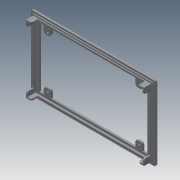
# Autodesk Inventor part: lower
Saved by Autodesk Inventor 2014 (Build 180170000, 170)
## iProperties
Created: 2014-09-06
Part Number: lower
Material: 一般
Document SubType Name: Modeling
Designer: Hideyuki Takei
Density: 1 g/cm^3
Appearance: 既定
Author: Hideyuki Takei
Autodesk Inventor part; units mm, degrees
ref_plane "YZ Plane" through (0, 0, 0) normal (1, 0, 0) x (0, 1, 0)
ref_plane "XZ Plane" through (0, 0, 0) normal (0, 1, 0) x (-1, 0, 0)
ref_plane "XY Plane" through (0, 0, 0) normal (0, 0, 1) x (1, 0, 0)
sketch "スケッチ2" plane through (0, 0, 0) normal (0, 1, 0) x (-1, 0, 0)
  line L0 (0, 0) -> (136, 0)
  line L1 (136, 0) -> (136, 81)
  line L2 (136, 81) -> (0, 81)
  line L3 (0, 81) -> (0, 0)
  dimension "d2" = 81
  dimension "d3" = 136
  constraints: 8 end point, 2 parallel, 1 horizontal, 1 perpendicular
  measures "d2" distance of L2.end L0.start
  measures "d3" distance of L1.end L2.end
extrude "押し出し1" add sketch "スケッチ2" along normal blind 2
sketch "スケッチ3" plane through (0, 0, 0) normal (0, 1, 0) x (-1, 0, 0)
  line L0 (5, 5) -> (131, 5)
  line L1 (131, 5) -> (131, 76)
  line L2 (131, 76) -> (5, 76)
  line L3 (5, 76) -> (5, 5)
  line L4 (136, 0) -> (136, 81) projected
  line L5 (136, 81) -> (0, 81) projected
  line L6 (132.5, 77.5) -> (126.5, 77.5)
  line L7 (126.5, 77.5) -> (126.5, 76)
  line L8 (126.5, 76) -> (132.5, 76)
  line L9 (132.5, 76) -> (132.5, 77.5)
  line L10 (131, 76) -> (132.5, 76)
  line L11 (132.5, 76) -> (132.5, 71)
  line L12 (132.5, 71) -> (131, 71)
  line L13 (131, 71) -> (131, 76)
  line L14 (131, 5) -> (132.5, 5)
  line L15 (132.5, 5) -> (132.5, 10)
  line L16 (132.5, 10) -> (131, 10)
  line L17 (131, 10) -> (131, 5)
  line L18 (132.5, 5) -> (126.5, 5)
  line L19 (126.5, 5) -> (126.5, 3.5)
  line L20 (126.5, 3.5) -> (132.5, 3.5)
  line L21 (132.5, 3.5) -> (132.5, 5)
  line L22 (5, 76) -> (3.5, 76)
  line L23 (3.5, 76) -> (3.5, 71)
  line L24 (3.5, 71) -> (5, 71)
  line L25 (5, 71) -> (5, 76)
  line L26 (3.5, 76) -> (9.5, 76)
  line L27 (9.5, 76) -> (9.5, 77.5)
  line L28 (9.5, 77.5) -> (3.5, 77.5)
  line L29 (3.5, 77.5) -> (3.5, 76)
  line L30 (5, 5) -> (3.5, 5)
  line L31 (3.5, 5) -> (3.5, 10)
  line L32 (3.5, 10) -> (5, 10)
  line L33 (5, 10) -> (5, 5)
  line L34 (3.5, 5) -> (9.5, 5)
  line L35 (9.5, 5) -> (9.5, 3.5)
  line L36 (9.5, 3.5) -> (3.5, 3.5)
  line L37 (3.5, 3.5) -> (3.5, 5)
  point P0 (0, 0)
  dimension "d6" = 126
  dimension "d7" = 71
  dimension "d8" = 5
  dimension "d9" = 5
  dimension "d10" = 1.5
  dimension "d11" = 1.5
  dimension "d12" = 5
  dimension "d13" = 6
  dimension "d14" = 0
  dimension "d17" = 1.5
  dimension "d18" = 1.5
  dimension "d19" = 6
  dimension "d20" = 5
  dimension "d21" = 5
  dimension "d22" = 1.5
  dimension "d23" = 1.5
  dimension "d24" = 6
  dimension "d25" = 6
  dimension "d26" = 1.5
  dimension "d27" = 1.5
  dimension "d28" = 5
  constraints: 72 end point, 18 parallel, 9 horizontal, 9 perpendicular, 1 point on line
  measures "d6" distance of L1.end L2.end
  measures "d7" distance of L0.end L1.end
  measures "d8" distance between parallel lines of L4 L1
  measures "d9" distance between parallel lines of L5 L2
  measures "d10" distance of L11.end L12.end
  measures "d11" distance of L8.end L6.start
  measures "d12" distance of L10.end L11.end
  measures "d13" distance of L6.start L6.end
  measures "d14" distance between parallel lines of L11 L9
  measures "d17" distance of L15.end L16.end
  measures "d18" distance of L20.end L14.end
  measures "d19" distance of L19.end L20.end
  measures "d20" distance of L14.end L15.end
  measures "d21" distance of L22.end L23.end
  measures "d22" distance of L23.end L24.end
  measures "d23" distance of L28.end L22.end
  measures "d24" distance of L27.end L28.end
  measures "d25" distance of L35.end L36.end
  measures "d26" distance of L34.end L35.end
  measures "d27" distance of L31.end L32.end
  measures "d28" distance of L30.end L31.end
extrude "押し出し2" add sketch "スケッチ3" against normal blind 9.01 contours L30 L31 L32 L3 | L0 L35 L36 L37 L30 | L0 L14 L21 L20 L19 | L24 L23 L22 L3 | L1 L16 L15 L14 | L22 L29 L28 L27 L2 | L1 L8 L11 L12 | L7 L6 L9 L8 L2
sketch "スケッチ5" plane through (0, 0, 0) normal (0, 1, 0) x (-1, 0, 0)
  line L0 (131, 76) -> (5, 76)
  line L1 (5, 76) -> (5, 5)
  line L2 (5, 5) -> (131, 5)
  line L3 (131, 5) -> (131, 76)
  line L4 (0, 81) -> (0, 0) projected
  line L5 (131, 76) -> (5, 76)
  line L6 (5, 76) -> (5, 77.5)
  line L7 (5, 77.5) -> (131, 77.5)
  line L8 (131, 77.5) -> (131, 76)
  line L9 (131, 5) -> (5, 5)
  line L10 (5, 5) -> (5, 3.5)
  line L11 (5, 3.5) -> (131, 3.5)
  line L12 (131, 3.5) -> (131, 5)
  line L13 (131, 77.5) -> (132.5, 77.5)
  line L14 (132.5, 77.5) -> (132.5, 3.5)
  line L15 (132.5, 3.5) -> (131, 3.5)
  line L16 (131, 3.5) -> (131, 77.5)
  line L17 (5, 77.5) -> (3.5, 77.5)
  line L18 (3.5, 77.5) -> (3.5, 3.5)
  line L19 (3.5, 3.5) -> (5, 3.5)
  line L20 (5, 3.5) -> (5, 77.5)
  dimension "d34" = 126
  dimension "d35" = 71
  dimension "d36" = 5
  dimension "d37" = 5
  dimension "d38" = 1.5
  dimension "d39" = 1.5
  dimension "d40" = 1.5
  dimension "d41" = 1.5
  dimension "d42" = 1.5
  dimension "d43" = 1.5
  constraints: 40 end point, 10 parallel, 5 horizontal, 5 perpendicular
  measures "d34" distance of L0.start L0.end
  measures "d35" distance of L2.end L0.start
  measures "d36" distance from line of L4.end L2
  measures "d37" distance between parallel lines of L4 L1
  measures "d38" distance of L5.end L6.end
  measures "d39" distance of L9.end L10.end
  measures "d40" distance of L14.end L15.end
  measures "d41" distance of L18.end L19.end
  measures "d42" distance between parallel lines of L19 L2
  measures "d43" distance between parallel lines of L18 L1
extrude "押し出し4" add sketch "スケッチ5" against normal blind 2 contours L8 L13 L14 L15 L12 L3 | L0 L6 L7 L8 | L1 L10 L19 L18 L17 L6 | L12 L11 L10 L2
sketch "スケッチ7" plane through (0, 0, 0) normal (0, 1, 0) x (-1, 0, 0)
  line L0 (9, 73.5) -> (127, 73.5)
  line L1 (127, 73.5) -> (127, 7.5)
  line L2 (127, 7.5) -> (9, 7.5)
  line L3 (9, 7.5) -> (9, 73.5)
  line L4 (136, 0) -> (136, 81) projected
  line L5 (136, 81) -> (0, 81) projected
  point P0 (0, 0)
  dimension "d50" = 66
  dimension "d51" = 118
  dimension "d52" = 9
  dimension "d53" = 7.5
  constraints: 8 end point, 2 parallel, 1 horizontal, 1 perpendicular
  measures "d50" distance of L0.end L1.end
  measures "d51" distance of L1.end L2.end
  measures "d52" distance between parallel lines of L1 L4
  measures "d53" distance between parallel lines of L5 L0
extrude "押し出し6" cut sketch "スケッチ7" along normal up to next
sketch "スケッチ9" plane through (-132.5, 0, 77.5) normal (0, 0, 1) x (1, 0, 0)
  line L0 (129, 0) -> (129, -9.01) projected
  line L1 (0, 0) -> (129, 0) projected
  line L2 (0, 0) -> (129, 0)
  line L3 (129, 0) -> (129, -1)
  line L4 (129, -1) -> (0, -1)
  line L5 (0, -1) -> (0, 0)
  point P0 (132.5, 0)
  dimension "d62" = 1
  constraints: 8 end point, 2 parallel, 1 horizontal, 1 perpendicular, 1 point on line
  measures "d62" distance of L4.end L1.start
extrude "押し出し8" add sketch "スケッチ9" along normal blind 1.5
sketch "スケッチ10" plane through (-3.5, 0, 3.5) normal (0, 0, -1) x (-1, 0, 0)
  line L0 (129, 0) -> (129, -9.01) projected
  line L1 (0, 0) -> (129, 0)
  line L2 (129, 0) -> (129, -1)
  line L3 (129, -1) -> (0, -1)
  line L4 (0, -1) -> (0, 0)
  point P0 (-3.5, 0)
  dimension "d65" = 1
  constraints: 8 end point, 2 parallel, 1 horizontal, 1 perpendicular, 1 point on line
  measures "d65" distance of L1.end L2.end
extrude "押し出し9" add sketch "スケッチ10" along normal blind 1.5
sketch "スケッチ11" plane through (-3.5, -9.01, 10) normal (1, 0, 0) x (0, 0, -1)
  line L0 (-69, 9.01) -> (8, 9.01)
  line L1 (8, 9.01) -> (8, 8.01)
  line L2 (8, 8.01) -> (-69, 8.01)
  line L3 (-69, 8.01) -> (-69, 9.01)
  point P0 (10, 9.01)
  constraints: 8 end point, 2 parallel, 1 horizontal, 1 perpendicular
extrude "押し出し10" add sketch "スケッチ11" along normal blind 1.5
sketch "スケッチ12" plane through (-132.5, -9.01, 3.5) normal (-1, 0, 0) x (0, 0, 1)
  line L0 (-1.5, 9.01) -> (75.5, 9.01)
  line L1 (75.5, 9.01) -> (75.5, 8.01)
  line L2 (75.5, 8.01) -> (-1.5, 8.01)
  line L3 (-1.5, 8.01) -> (-1.5, 9.01)
  point P0 (-3.5, 9.01)
  constraints: 8 end point, 2 parallel, 1 horizontal, 1 perpendicular
extrude "押し出し11" add sketch "スケッチ12" along normal blind 1.5
sketch "スケッチ13" plane through (0, 2, 0) normal (0, 1, 0) x (1, 0, 0)
  line L0 (-127, -7.5) -> (-9, -7.5) projected
  line L1 (-9, -7.5) -> (-9, -73.5) projected
  line L2 (-9, -73.5) -> (-127, -73.5) projected
  line L3 (-9, -73.5) -> (-127, -73.5) projected
  line L4 (-127, -73.5) -> (-127, -7.5) projected
  line L5 (-127, -7.5) -> (-9, -7.5) projected
  line L6 (-122, -7.5) -> (-114, -7.5)
  line L7 (-114, -7.5) -> (-114, -15.5)
  line L8 (-114, -15.5) -> (-122, -15.5)
  line L9 (-122, -15.5) -> (-122, -7.5)
  line L10 (-122, -73.5) -> (-114, -73.5)
  line L11 (-114, -73.5) -> (-114, -65.5)
  line L12 (-114, -65.5) -> (-122, -65.5)
  line L13 (-122, -65.5) -> (-122, -73.5)
  line L14 (-14, -7.5) -> (-22, -7.5)
  line L15 (-22, -7.5) -> (-22, -15.5)
  line L16 (-22, -15.5) -> (-14, -15.5)
  line L17 (-14, -15.5) -> (-14, -7.5)
  line L18 (-14, -73.5) -> (-22, -73.5)
  line L19 (-22, -73.5) -> (-22, -65.5)
  line L20 (-22, -65.5) -> (-14, -65.5)
  line L21 (-14, -65.5) -> (-14, -73.5)
  circle A0 centre (-118, -12.5) radius 1.25
  circle A1 centre (-118, -68.5) radius 1.25
  circle A2 centre (-18, -12.5) radius 1.25
  circle A3 centre (-18, -68.5) radius 1.25
  point P0 (-44.5213, -7.5)
  point P1 (-44.5213, -73.5)
  point P2 (-91.4787, -7.5)
  point P3 (-91.4787, -73.5)
  dimension "d72" = 8
  dimension "d73" = 8
  dimension "d74" = 8
  dimension "d75" = 8
  dimension "d76" = 8
  dimension "d77" = 8
  dimension "d78" = 8
  dimension "d79" = 8
  dimension "d80" = 5
  dimension "d81" = 5
  dimension "d82" = 5
  dimension "d83" = 5
  dimension "d84" = 2.5
  dimension "d85" = 2.5
  dimension "d86" = 2.5
  dimension "d87" = 2.5
  dimension "d88" = 4
  dimension "d89" = 3
  dimension "d90" = 3
  dimension "d91" = 4
  dimension "d92" = 4
  dimension "d93" = 5
  dimension "d94" = 4
  dimension "d95" = 5
  constraints: 32 end point, 8 parallel, 4 centre point, 4 horizontal, 4 perpendicular, 4 point on line
  measures "d72" distance of L8.end L6.start
  measures "d73" distance of L12.end L10.start
  measures "d74" distance of L20.end L18.start
  measures "d75" distance of L16.end L14.start
  measures "d76" distance of L7.end L8.end
  measures "d77" distance of L11.end L12.end
  measures "d78" distance of L19.end L20.end
  measures "d79" distance of L15.end L16.end
  measures "d80" distance between parallel lines of L9 L4
  measures "d81" distance between parallel lines of L4 L13
  measures "d82" distance between parallel lines of L1 L17
  measures "d83" distance between parallel lines of L1 L21
  measures "d84" diameter of A3
  measures "d85" diameter of A1
  measures "d86" diameter of A0
  measures "d87" diameter of A2
  measures "d88" distance from line of L9 A0.centre
  measures "d89" distance from line of L8 A0.centre
  measures "d90" distance from line of L16 A2.centre
  measures "d91" distance from line of L15 A2.centre
  measures "d92" distance from line of L19 A3.centre
  measures "d93" distance from line of L2 A3.centre
  measures "d94" distance from line of L13 A1.centre
  measures "d95" distance from line of L3 A1.centre
extrude "押し出し12" add sketch "スケッチ13" against normal blind 2 contours L0 L7 L8 L9 | L13 L12 L11 L2 | L0 L17 L16 L15 | L19 L20 L21 L2
fillet "フィレット1" radius 3 8 edges at (-14, 1, 65.5) (-22, 1, 65.5) (-114, 1, 65.5) (-122, 1, 65.5) (-114, 1, 15.5) (-122, 1, 15.5) (-14, 1, 15.5) (-22, 1, 15.5)
fillet "フィレット2" radius 1.5 8 edges at (0, 1, 81) (0, 1, 0) (-136, 1, 0) (-136, 1, 81) (-134, -0.5, 79) (-134, -0.5, 2) (-2, -0.5, 2) (-2, -0.5, 79)
sketch "スケッチ15" plane through (0, -2, 0) normal (0, -1, 0) x (1, 0, 0)
  line L0 (-101.5, 77.5) -> (-101.5, 76) projected
  line L1 (-126.5, 76) -> (-9.5, 76) projected
  line L2 (-9.5, 77.5) -> (-126.5, 77.5) projected
  line L3 (-93, 77.5) -> (-43, 77.5)
  line L4 (-43, 77.5) -> (-43, 76)
  line L5 (-43, 76) -> (-93, 76)
  line L6 (-93, 76) -> (-93, 77.5)
  point P0 (-34.5, 76)
  point P1 (-34.5, 77.5)
  point P2 (0, 0)
  dimension "d107" = 50
  dimension "d108" = 8.5
  constraints: 8 end point, 2 parallel, 2 point on line, 1 horizontal, 1 perpendicular
  measures "d107" distance of L3.start L3.end
  measures "d108" distance from line of L0 L5.end
extrude "押し出し14" [suppressed]
fillet "フィレット4" radius 2 8 edges at (-131.75, -9.01, 71) (-131.75, -9.01, 10) (-126.5, -9.01, 4.25) (-4.25, -9.01, 71) (-4.25, -9.01, 10) (-9.5, -9.01, 4.25) (-126.5, -9.01, 76.75) (-9.5, -9.01, 76.75)
equation "\"d52\" = 0.5 * d3 - 0.5 * d51"
equation "\"d53\" = 0.5 * d2 - 0.5 * d50"
